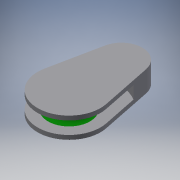
# Autodesk Inventor part: katrol
Saved by Autodesk Inventor 2017 (Build 210142000, 142)
## iProperties
Created: 2017-02-22
Part Number: katrol
Material: Generic
Document SubType Name: Modeling
Designer: user
Density: 1 g/cm^3
Appearance: Default
Author: user
Autodesk Inventor part; units mm, degrees
ref_plane "YZ Plane" through (0, 0, 0) normal (1, 0, 0) x (0, 1, 0)
ref_plane "XZ Plane" through (0, 0, 0) normal (0, 1, 0) x (-1, 0, 0)
ref_plane "XY Plane" through (0, 0, 0) normal (0, 0, 1) x (1, 0, 0)
sketch "Sketch1" plane through (0, 0, 0) normal (0, 0, 1) x (1, 0, 0)
  arc A0 (-29.3939, 6) -> (29.3939, 6) centre (0, 0) ccw
  line L0 (-29.3939, 6) -> (-19.5959, 54)
  arc A1 (19.5959, 54) -> (-19.5959, 54) centre (0, 50) ccw
  line L1 (19.5959, 54) -> (29.3939, 6)
  dimension "d0" = 30
  dimension "d1" = 50
  dimension "d2" = 20
  constraints: 4 end point, 4 point on circle, 3 tangent, 2 centre point, 1 coincident, 1 horizontal alignment, 1 vertical alignment
  measures "d0" radius of A0
  measures "d1" distance of point (0, 0) A1.centre
  measures "d2" radius of A1
extrude "Extrusion1" add sketch "Sketch1" along normal mid plane 20
sketch "Sketch2" plane through (0, 0, 0) normal (1, 0, 0) x (0, 1, 0)
  line L0 (6, -10) -> (6, 10) projected
  line L1 (6, 10) -> (6, 10) projected
  line L2 (6, 10) -> (6, -10) projected
  line L3 (6, -10) -> (6, -10) projected
  line L4 (6, 10) -> (6, -10) projected
  line L5 (54, 10) -> (6, 10) projected
  line L6 (54, -10) -> (54, 10) projected
  line L7 (6, -10) -> (54, -10) projected
  line L8 (0, 26.5317) -> (0, -26.5317)
  line L9 (45, 6) -> (20, 6)
  arc A0 (20, 6) -> (20, -6) centre (20, 0) ccw
  line L10 (20, -6) -> (45, -6)
  line L11 (45, -6) -> (45, 6)
  point P0 (0, 0)
  point P1 (0, 0)
  dimension "d5" = 53.0634
  dimension "d6" = 40
  dimension "d7" = 12
  dimension "d8" = 90
  constraints: 8 end point, 2 horizontal, 2 point on circle, 2 tangent, 1 centre point, 1 coincident, 1 horizontal alignment, 1 midpoint, 1 perpendicular, 1 vertical
  measures "d5" distance of L8.start L8.end
  measures "d6" diameter of A0.centre L8
  measures "d7" distance of L10.end L9.start
  measures "d8" diameter of L11 L8
revolve "Revolution1" cut sketch "Sketch2" angle 360 about axis through (0, 0, 26.5317) along (0, 0, -1) contours L11 L10 A0 L9
body "Solid1"
